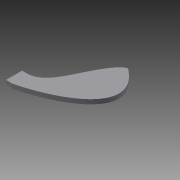
# Autodesk Inventor part: cola
Saved by Autodesk Inventor 2015 (Build 190159000, 159)
## iProperties
Created: 2017-11-29
Part Number: cola
Material: Generic
Document SubType Name: Modeling
Designer: Max
Density: 1 g/cm^3
Appearance: Default
Author: Max
Autodesk Inventor part; units mm, degrees
ref_plane "YZ Plane" through (0, 0, 0) normal (1, 0, 0) x (0, 1, 0)
ref_plane "XZ Plane" through (0, 0, 0) normal (0, 1, 0) x (-1, 0, 0)
ref_plane "XY Plane" through (0, 0, 0) normal (0, 0, 1) x (1, 0, 0)
sketch "Sketch1" plane through (0, 0, 0) normal (0, 0, 1) x (1, 0, 0)
  line L0 (0, 0) -> (8, 0)
  line L1 (8, 20) -> (0, 20)
  line L2 (0, 20) -> (0, 0)
  line L3 (8, 0) -> (49.9131, 10) construction
  line L4 (49.9131, 10) -> (120.5614, 44.2415) construction
  line L5 (120.5614, 44.2415) -> (63.5038, 88.1716) construction
  spline S0 degree 3 poles (8, 0) (49.9131, 10) (120.5614, 44.2415) (63.5038, 88.1716) knots 1 1 1 1 2 2 2 2
  line L6 (8, 20) -> (35.2198, 23.4351) construction
  line L7 (35.2198, 23.4351) -> (35.2198, 60.333) construction
  line L8 (35.2198, 60.333) -> (55.6473, 88.1716) construction
  line L9 (55.6473, 88.1716) -> (63.5038, 88.1716) construction
  spline S1 degree 4 poles (8, 20) (35.2198, 23.4351) (35.2198, 60.333) (55.6473, 88.1716) (63.5038, 88.1716) knots 1 1 1 1 1 2 2 2 2 2
  dimension "d6" = 8
  constraints: 6 end point, 2 horizontal, 1 parallel, 1 vertical, 6 other
  measures "d6" distance of L1.start L1.end
extrude "Extrusion1" add sketch "Sketch1" along normal blind 5.5
body "Solid1"
